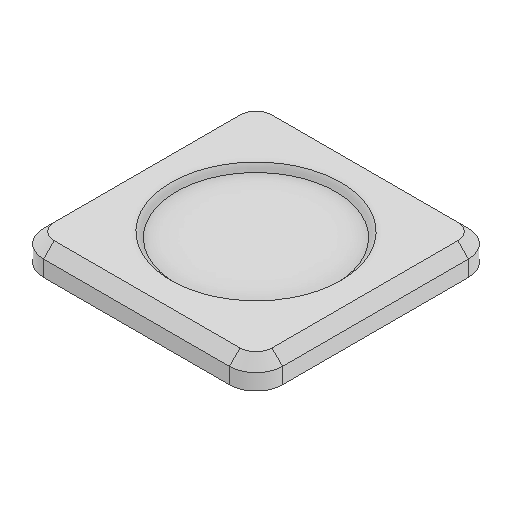
# Autodesk Inventor part: Top
Saved by Autodesk Inventor 2025.2 (Build 292293000, 293)
## iProperties
Created: 2025-03-03
Part Number: Top
Material: Generic
Document SubType Name: Modeling
Designer: Marcu
Density: 1 g/cm^3
Appearance: Default
Author: Marcu
Autodesk Inventor part; units mm, degrees
ref_plane "YZ Plane" through (0, 0, 0) normal (1, 0, 0) x (0, 1, 0)
ref_plane "XZ Plane" through (0, 0, 0) normal (0, 1, 0) x (-1, 0, 0)
ref_plane "XY Plane" through (0, 0, 0) normal (0, 0, 1) x (1, 0, 0)
sketch "Sketch1" plane through (0, 0, 0) normal (0, 0, 1) x (1, 0, 0)
  line L0 (-22.5, 22.5) -> (22.5, 22.5)
  line L1 (22.5, 22.5) -> (22.5, -22.5)
  line L2 (22.5, -22.5) -> (-22.5, -22.5)
  line L3 (-22.5, -22.5) -> (-22.5, 22.5)
  point P0 (0, 0)
  dimension "d0" = 45
  dimension "d1" = 45
  dimension "d2" = 22.5
  dimension "d3" = 22.5
  constraints: 8 end point, 2 parallel, 1 horizontal, 1 perpendicular
  measures "d0" distance between parallel lines of L3 L1
  measures "d1" distance between parallel lines of L2 L0
  measures "d2" distance from line of point (0, 0) L1
  measures "d3" distance from line of point (0, 0) L2
extrude "Extrusion1" add sketch "Sketch1" along normal blind 5
fillet "Fillet1" radius 5 4 edges at (-22.5, -22.5, 2.5) (22.5, -22.5, 2.5) (22.5, 22.5, 2.5) (-22.5, 22.5, 2.5)
sketch "Sketch2" plane through (0, 0, 5) normal (0, 0, 1) x (1, 0, 0)
  circle A0 centre (0, 0) radius 15
  dimension "d7" = 30
  constraints: 1 centre point, 1 coincident
  measures "d7" diameter of A0
extrude "Extrusion2" cut sketch "Sketch2" against normal blind 1
chamfer "Chamfer1" distance 2 angle 45 8 edges at (0, -22.5, 5) (21.0355, -21.0355, 5) (22.5, 0, 5) (21.0355, 21.0355, 5) (0, 22.5, 5) (-21.0355, 21.0355, 5) (-22.5, 0, 5) (-21.0355, -21.0355, 5)
sketch "Sketch3" plane through (0, 0, 0) normal (0, 0, -1) x (-1, 0, 0)
  circle A0 centre (-16.25, 0) radius 2.5
  circle A1 centre (16.25, 0) radius 2.5
  point P0 (0, 0)
  point P1 (0, 0)
  dimension "d13" = 5
  constraints: 2 centre point
  measures "d13" diameter of A0
extrude "Extrusion3" add sketch "Sketch3" along normal blind 3
chamfer "Chamfer2" distance 1 angle 45 1 edges at (-15, 0, 5)
body "Solid1"
